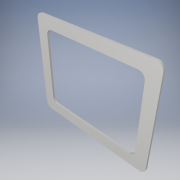
# Autodesk Inventor part: Display Bezel
Saved by Autodesk Inventor 2019 (Build 230136000, 136)
## iProperties
Created: 2019-03-08
Part Number: Display Bezel
Material: Aluminum 6061
Document SubType Name: Modeling
Designer: Jackson Smith
Density: 2.7 g/cm^3
Appearance: Aluminum - Flat
Author: Jackson Smith
Autodesk Inventor part; units mm, degrees
ref_plane "YZ Plane" through (0, 0, 0) normal (1, 0, 0) x (0, 1, 0)
ref_plane "XZ Plane" through (0, 0, 0) normal (0, 1, 0) x (-1, 0, 0)
ref_plane "XY Plane" through (0, 0, 0) normal (0, 0, 1) x (1, 0, 0)
sketch "Sketch1" plane through (0, 0, 0) normal (0, 0, 1) x (1, 0, 0)
  line L0 (-13, 10) -> (13, 10)
  line L1 (13, 10) -> (13, -10)
  line L2 (13, -10) -> (-13, -10)
  line L3 (-13, -10) -> (-13, 10)
  line L4 (-13, 10) -> (13, -10) construction
  line L5 (13, 10) -> (-13, -10) construction
  line L6 (-16, 13) -> (16, 13)
  line L7 (16, 13) -> (16, -13)
  line L8 (16, -13) -> (-16, -13)
  line L9 (-16, -13) -> (-16, 13)
  line L10 (-16, 13) -> (16, -13) construction
  line L11 (16, 13) -> (-16, -13) construction
  point P0 (0, 0)
  dimension "d0" = 26
  dimension "d1" = 20
  dimension "d2" = 3
  dimension "d3" = 3
  constraints: 24 end point, 4 midpoint, 4 parallel, 2 horizontal, 2 perpendicular
  measures "d0" distance of L1.end L2.end
  measures "d1" distance of L0.end L1.end
  measures "d2" distance between parallel lines of L0 L6
  measures "d3" distance between parallel lines of L9 L3
extrude "Extrusion1" add sketch "Sketch1" along normal blind 0.508
fillet "Fillet1" radius 1.5875 8 edges at (-13, 10, 0.254) (-13, -10, 0.254) (13, -10, 0.254) (13, 10, 0.254) (16, -13, 0.254) (16, 13, 0.254) (-16, 13, 0.254) (-16, -13, 0.254)
body "Solid1"
